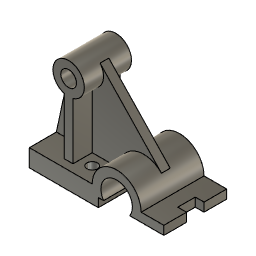
Sketch21_Final v1 (Autodesk Fusion 360 design; units mm, degrees)
Autodesk Fusion 360 part; units mm, degrees
sketch "Sketch1" plane through (0, 0, 0) normal (0, 1, 0) x (1, 0, 0)
  line L0 (0, 0) -> (-36, 0)
  line L1 (-36, 0) -> (-36, 20)
  circle A0 centre (0, -82) radius 9
  circle A1 centre (0, -82) radius 18
  line L2 (0, 0) -> (36, 0)
  line L3 (82, 0) -> (118, 0)
  line L4 (118, 0) -> (118, 10)
  line L5 (118, 10) -> (78.9666, 10)
  line L6 (49.0334, 10) -> (43.0334, 10)
  line L7 (43.0334, 10) -> (43.0334, 20)
  line L8 (-36, 20) -> (44.4041, 20)
  arc A2 (44.4041, 20) -> (90.1534, 10) centre (64, 0) ccw
  arc A3 (49.0334, 10) -> (78.9666, 10) centre (64, 0) ccw
  line L9 (12.0259, -95.3932) -> (84.3038, -19.281)
  line L10 (-36, 0) -> (-17.5996, -85.7754)
  line L11 (0, 0) -> (5, 0)
  line L12 (5, 0) -> (5, -64.7084)
  line L13 (0, 0) -> (-5, 0)
  line L14 (-5, 0) -> (-5, -64.7084)
  dimension "d1" = 36
  dimension "d2" = 20
  dimension "d4" = 82
  dimension "d5" = 18
  dimension "d6" = 36
  dimension "d7" = 64
  dimension "d8" = 36
  dimension "d9" = 56
  dimension "d12" = 54
  dimension "d13" = 10
  dimension "d14" = 6
  dimension "d15" = 10
  dimension "d22" = 5
  dimension "d23" = 64.7084
  dimension "d24" = 5
  constraint coincident L0.start L2.start
  constraint horizontal L0
  constraint perpendicular L0 L1
  constraint perpendicular L1 L8
  constraint concentric A0 A1
  constraint parallel L0 L2
  constraint concentric A2 A3
  constraint parallel L2 L3
  constraint perpendicular L3 L4
  constraint perpendicular L4 L5
  constraint parallel L5 L6
  constraint coincident L7.end L8
  constraint perpendicular L7 L8
  constraint coincident A3 L3.start
  constraint coincident L5 A2.end
  constraint coincident A2 L2.end
  constraint coincident A1 L9.start
  constraint coincident A2 L9.end
  constraint tangent A2 L9
  constraint coincident A1 L10.end
  constraint tangent A1 L10
  constraint parallel L2 L11
  constraint coincident A1 L12.end
  constraint perpendicular L2 L12
  constraint parallel L0 L13
  constraint coincident A1 L14.end
  constraint perpendicular L13 L14
  measures "d1" distance of L0.start L0.end
  measures "d2" distance of L0.end L1.end
  measures "d4" distance of L0.start A0.centre
  measures "d5" diameter of A0
  measures "d6" diameter of A1
  measures "d7" distance of L0.start A2.centre
  measures "d8" diameter of A3
  measures "d9" diameter of A2
  measures "d12" distance of A2.centre L3.end
  measures "d13" distance of L3.end L4.end
  measures "d14" distance of L6.start L6.end
  measures "d15" distance of L6.end L7.end
  measures "d22" distance of L0.start L11.end
  measures "d23" distance of L11.end L12.end
  measures "d24" distance of L0.start L13.end
extrude "Extrude1" add sketch "Sketch1" along normal mid plane 72 contours L0 L1 L2 L7 L8 A2 L11 L13 | L3 L6 L7 A2 A3 | L3 L4 L5 A2 | L3 L5 A2 A3 makes body 1
extrude "Extrude2" add sketch "Sketch1" along normal mid plane 54 separate body contours A1 L9 | A1 L9 makes body 2
extrude "Extrude3" add sketch "Sketch1" along normal mid plane 54 contours L0 A1 L2 L11 L12 L13 L14 bodies 2
extrude "Extrude4" add sketch "Sketch1" along normal mid plane 10 contours L0 A1 L10 L14 bodies 1 2
extrude "Extrude5" add sketch "Sketch1" along normal mid plane 10 contours A1 L2 A2 L9 L12 bodies 1
sketch "Sketch4" plane through (0, 0, 0) normal (0, 0, 1) x (1, 0, 0)
  line L0 (0, 0) -> (18, 0)
  line L1 (108, -10) -> (128, -10)
  line L2 (128, -10) -> (128, 10)
  line L3 (128, 10) -> (108, 10)
  line L4 (108, 10) -> (108, -10)
  line L5 (108, -10) -> (128, 10) construction
  line L6 (128, -10) -> (108, 10) construction
  point P0 (118, 0)
  dimension "d31" = 18
  dimension "d40" = 20
  dimension "d41" = 20
  constraint coincident L0.start origin
  constraint horizontal L0
  constraint horizontal L1
  constraint perpendicular L1 L2
  constraint parallel L1 L3
  constraint parallel L2 L4
  constraint coincident L5 P0
  constraint coincident L6 P0
  measures "d31" distance of L0.start L0.end
  measures "d40" distance of L2.end L3.end
  measures "d41" distance of L1.end L2.end
hole "Hole1" at (18.0126, -18.0267, 0) direction (0, 0, -1) diameter 12 depth 30 tip angle 118 bodies 1
hole "Hole2" at (17.8831, 17.9931, 0) direction (0, 0, -1) diameter 12 depth 30 tip angle 118 bodies 1
extrude "Extrude6" cut sketch "Sketch4" against normal blind 20 bodies 1
